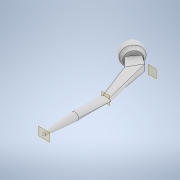
# Autodesk Inventor part: ProtesiAnca
Saved by Autodesk Inventor 2020.5 (Build 245400000, 400)
## iProperties
Created: 2022-07-05
Part Number: ProtesiAnca
Material: Generico
Document SubType Name: Modeling
Designer: Utente
Density: 1 g/cm^3
Appearance: Default
Author: Utente
Autodesk Inventor part; units mm, degrees
ref_plane "YZ Plane" through (0, 0, 0) normal (1, 0, 0) x (0, 1, 0)
ref_plane "XZ Plane" through (0, 0, 0) normal (0, 1, 0) x (-1, 0, 0)
sketch "Schizzo1" plane through (0, 0, 0) normal (0, 0, 1) x (1, 0, 0)
  circle A0 centre (0, 0) radius 6.05
  dimension "d0" = 12.1
  constraints: 1 centre point, 1 coincident
  measures "d0" diameter of A0
ref_plane "Piano di lavoro1" through (0, 0, -50) normal (0, 0, 1) x (1, 0, 0)
sketch "Schizzo3" plane through (0, 0, -50) normal (0, 0, 1) x (1, 0, 0)
  ellipse E0 centre (0, 0) end of major axis (8, 0) minor radius 2.417202
  dimension "d3" = 8
  constraints: 1 centre point, 1 coincident, 1 other
loft "Loft1" add profiles "Schizzo1", "Schizzo3"
ref_plane "Piano di lavoro2" through (0, 0, 50) normal (0, 0, 1) x (1, 0, 0)
sketch "Schizzo5" plane through (0, 0, 50) normal (0, 0, 1) x (1, 0, 0)
  line L0 (0, 0) -> (2.5, 0)
  line L1 (0, 0) -> (-2.5, 0)
  arc A0 (2.5, 0) -> (-2.5, 0) centre (0, 0) ccw
  dimension "d12" = 2.5
  dimension "d13" = 2.5
  dimension "d14" = 2.5
  constraints: 4 end point, 2 horizontal, 2 point on circle, 1 centre point
  measures "d12" distance of L0.start L0.end
  measures "d13" distance of L0.start L1.end
  measures "d14" radius of A0
revolve "Rivoluzione1" add sketch "Schizzo5" angle 180 about axis through (0, 0, 50) along (1, 0, 0)
loft "Loft2" add section 1 edges at (0, 2.5, 50) (0, -2.5, 50) section 2 edges at (-6.05, 0, 0)
sketch "Schizzo7" plane through (0, 0, 0) normal (0, 1, 0) x (-1, 0, 0)
  line L0 (-6.05, 0) -> (-8, -50)
  line L1 (-8, -50) -> (-8, -125)
  line L2 (-8, -125) -> (12, -125)
  line L3 (12, -125) -> (26.483919, -134.775898)
  line L4 (26.483919, -134.775898) -> (39.406492, -119.793204)
  line L5 (39.406492, -119.793204) -> (23.674663, -104.061374)
  line L6 (-8, -50) -> (8, -50)
  arc A0 (8, -50) -> (23.674663, -104.061374) centre (128.092499, -44.483198) ccw
  line L7 (8, -50) -> (-8, -50)
  line L8 (0, -50) -> (0, -125)
  line L9 (23.674663, -104.061374) -> (12, -125)
  point P0 (0, 0)
  dimension "d20" = 75
  dimension "d21" = 20
  constraints: 16 end point, 2 horizontal, 2 point on circle, 1 centre point, 1 midpoint, 1 perpendicular, 1 point on line, 1 vertical
  measures "d20" distance of L0.end L1.end
  measures "d21" distance of L1.end L2.end
extrude "Estrusione1" add sketch "Schizzo7" along normal mid plane 10 contours L9 L5 L4 L3
ref_plane "Piano di lavoro3" through (0, 0, -125) normal (0, 0, 1) x (1, 0, 0)
loft "Loft3" add section 1 edges at (-12, 0, -125) (-17.837332, 5, -114.530687) (-23.674663, 0, -104.061374) (-17.837332, -5, -114.530687) section 2 edges at (-8, 0, -50)
sketch "Schizzo11" plane through (0, 0, 0) normal (0, 1, 0) x (-1, 0, 0)
  line L0 (26.483919, -134.775898) -> (39.406492, -119.793204)
  line L1 (32.945205, -127.284551) -> (54.485655, -143.563649)
  line L2 (32.945205, -127.284551) -> (59.945205, -127.284551) construction
  line L3 (32.945205, -127.284551) -> (24.900904, -136.611277)
  arc A0 (28.024206, -143.26834) -> (54.485655, -143.563649) centre (41.357099, -134.261075) ccw
  arc A1 (28.024206, -143.26834) -> (24.900904, -136.611277) centre (21.88154, -142.089089) ccw
  point P0 (0, 0)
  dimension "d30" = 27
  dimension "d31" = 37.08
  constraints: 6 end point, 4 point on circle, 2 centre point, 1 equal length, 1 horizontal, 1 midpoint
  measures "d30" distance of L1.start L1.end
  measures "d31" angle of L1 L2
revolve "Rivoluzione2" add sketch "Schizzo11" angle 360 about axis through (-32.945205, 0, -127.284551) along (-0.7977944, 0, -0.6029295)
